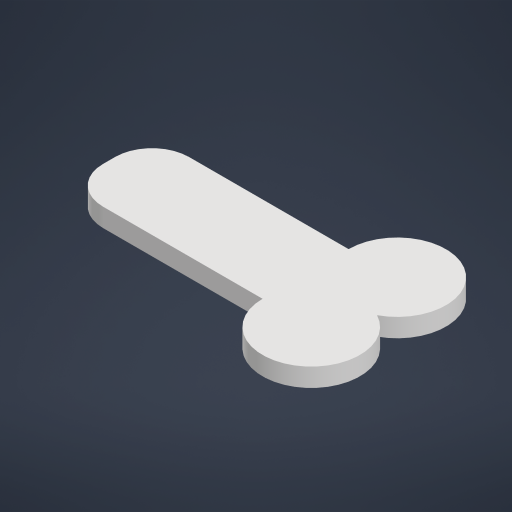
# Autodesk Inventor part: Part1
Saved by Autodesk Inventor 2023 (Build 270158000, 158)
## iProperties
Created: 2022-11-12
Part Number: Part1
Material: Generic
Document SubType Name: Modeling
Designer: jevan
Density: 1 g/cm^3
Appearance: Default
Author: jevan
Autodesk Inventor part; units mm, degrees
ref_plane "YZ Plane" through (0, 0, 0) normal (1, 0, 0) x (0, 1, 0)
ref_plane "XZ Plane" through (0, 0, 0) normal (0, 1, 0) x (-1, 0, 0)
ref_plane "XY Plane" through (0, 0, 0) normal (0, 0, 1) x (1, 0, 0)
sketch "Sketch1" plane through (0, 0, 0) normal (0, 1, 0) x (-1, 0, 0)
  line L0 (0, 0) -> (16.8248, 0)
  line L1 (16.8248, 0) -> (16.8248, -5.9031)
  line L2 (16.8248, -5.9031) -> (0, -5.9031)
  line L3 (0, -5.9031) -> (0, 0)
  circle A0 centre (0, 0) radius 3.3405
  line L4 (16.8248, -2.9515) -> (0, -2.9515)
  circle A1 centre (0, -5.9031) radius 3.3405
  point P0 (3.3405, 0)
  point P1 (-1.5644, -2.9515)
  point P2 (3.3405, -5.9031)
  constraints: 10 end point, 2 centre point, 2 midpoint, 2 parallel, 1 coincident, 1 horizontal, 1 perpendicular, 1 symmetric about line, 1 other
extrude "Extrusion1" add sketch "Sketch1" along normal blind 1.27
fillet "Fillet1" radius 2.54 2 edges at (-16.8248, 0.635, 0) (-16.8248, 0.635, -5.9031)
body "Solid1"
